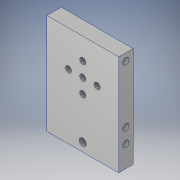
# Autodesk Inventor part: Hook Part
Saved by Autodesk Inventor 2019.4 (Build 234330000, 330)
## iProperties
Created: 2020-03-10
Part Number: Hook Part
Material: Aluminum 6061
Document SubType Name: Modeling
Designer: admin
Density: 2.7 g/cm^3
Appearance: Aluminum - Flat
Author: admin
Autodesk Inventor part; units mm, degrees
ref_plane "YZ Plane" through (0, 0, 0) normal (1, 0, 0) x (0, 1, 0)
ref_plane "XZ Plane" through (0, 0, 0) normal (0, 1, 0) x (-1, 0, 0)
ref_plane "XY Plane" through (0, 0, 0) normal (0, 0, 1) x (1, 0, 0)
sketch "Sketch1" plane through (0, 0, 0) normal (0, 0, 1) x (1, 0, 0)
  line L0 (-25, -35) -> (25, -35)
  line L1 (25, -35) -> (25, 35)
  line L2 (25, 35) -> (-25, 35)
  line L3 (-25, 35) -> (-25, -35)
  line L4 (-25, -35) -> (25, 35) construction
  line L5 (25, -35) -> (-25, 35) construction
  circle A0 centre (0, -29) radius 2.5
  line L6 (-10, 10) -> (10, 10) construction
  line L7 (0, 0) -> (0, 20) construction
  circle A1 centre (-10, 10) radius 2.1
  circle A2 centre (0, 20) radius 2.1
  circle A3 centre (10, 10) radius 2.1
  circle A4 centre (0, 0) radius 2.1
  circle A5 centre (0, 10) radius 2.1
  point P0 (0, 0)
  point P1 (0, 0)
  point P2 (0, 0)
  point P3 (0, 35)
  dimension "d0" = 5
  dimension "d8" = 50
  dimension "d9" = 70
  dimension "d10" = 6
  dimension "d11" = 20
  dimension "d12" = 20
  dimension "d13" = 4.2
  dimension "d14" = 4.2
  dimension "d15" = 4.2
  dimension "d16" = 4.2
  dimension "d17" = 25
  dimension "d28" = 4.2
  constraints: 16 end point, 7 midpoint, 6 centre point, 5 coincident, 2 horizontal, 2 parallel, 2 point on line, 1 perpendicular, 1 vertical
  measures "d0" diameter of A0
  measures "d8" distance of L1.end L2.end
  measures "d9" distance of L0.end L1.end
  measures "d10" distance from line of L0 A0.centre
  measures "d11" distance of L7.start L7.end
  measures "d12" distance of L6.start L6.end
  measures "d13" diameter of A1
  measures "d14" diameter of A2
  measures "d15" diameter of A3
  measures "d16" diameter of A4
  measures "d17" distance between parallel lines of L2 L6
  measures "d28" diameter of A5
extrude "Extrusion1" add sketch "Sketch1" along normal blind 10
sketch "Sketch2" plane through (25, -35, 0) normal (1, 0, 0) x (0, 0, -1)
  circle A0 centre (-5, 65) radius 2.2
  circle A1 centre (-5, 15) radius 2.2
  line L0 (-5, 15) -> (-5, 65) construction
  line L1 (0, 70) -> (-10, 70) projected
  line L2 (0, 0) -> (-10, 0) projected
  circle A2 centre (-5, 25) radius 2.2
  point P0 (0, 35)
  point P1 (-5, 70)
  dimension "d20" = 4.4
  dimension "d21" = 4.4
  dimension "d22" = 5
  dimension "d23" = 15
  dimension "d24" = 4.4
  dimension "d25" = 10
  constraints: 3 centre point, 2 end point, 2 point on line, 1 midpoint, 1 vertical
  measures "d20" diameter of A0
  measures "d21" diameter of A1
  measures "d22" distance from line of L1 L0.end
  measures "d23" distance from line of L2 L0.start
  measures "d24" diameter of A2
  measures "d25" distance of L0.start A2.centre
extrude "Extrusion2" cut sketch "Sketch2" against normal through all
body "Solid1"
